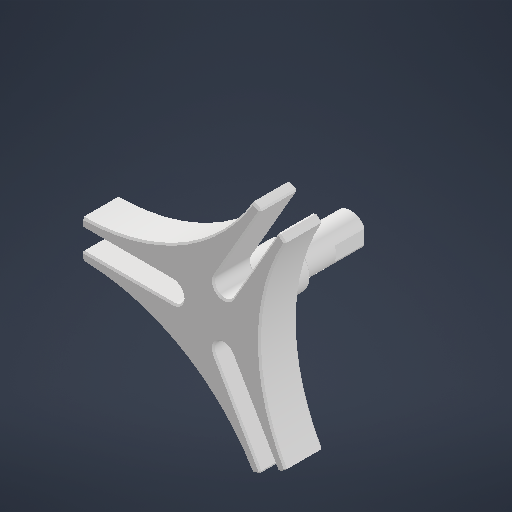
# Autodesk Inventor part: Geneva2_Output
Saved by Autodesk Inventor 2026.3 (Build 303398000, 398)
## iProperties
Created: 2026-05-01
Part Number: Geneva2_Output
Material: Generic
Document SubType Name: Modeling
Designer: frede
Density: 1 g/cm^3
Appearance: Default
Author: frede
Autodesk Inventor part; units mm, degrees
ref_plane "YZ Plane" through (0, 0, 0) normal (1, 0, 0) x (0, 1, 0)
ref_plane "XZ Plane" through (0, 0, 0) normal (0, 1, 0) x (-1, 0, 0)
ref_plane "XY Plane" through (0, 0, 0) normal (0, 0, 1) x (1, 0, 0)
sketch "Sketch2" plane through (0, 0, 0) normal (0, 0, 1) x (1, 0, 0)
  line L0 (0, 0) -> (10, 17.3205)
  line L1 (0, 0) -> (20, 0) construction
  line L2 (10, 17.3205) -> (40, 0)
  line L3 (0, 0) -> (40, 0)
  circle A0 centre (0, 0) radius 20
  circle A1 centre (40, 0) radius 34.641
  circle A2 centre (0, 0) radius 5.359
  arc A3 (1.2939, 5.441) -> (4.0651, 3.841) centre (2.6795, 4.641) ccw
  line L4 (8.4, 17.3205) -> (8.4, 0)
  arc A4 (8.4, 0) -> (12.518, -15.5981) centre (40, 0) ccw
  arc A5 (12.518, 15.5981) -> (8.4, 0) centre (40, 0) ccw
  arc A6 (12.518, -15.5981) -> (12.518, 15.5981) centre (40, 0) ccw
  line L5 (1.2939, 5.441) -> (8.6144, 18.1205)
  line L6 (11.3856, 16.5205) -> (4.0651, 3.841)
  arc A7 (11.3525, 16.4657) -> (8.5835, 18.0644) centre (10, 17.3205) ccw
  arc A8 (-19.7673, 3.0419) -> (-4.2, 7.2746) centre (-20, 34.641) ccw
  line L7 (-20, 1.6) -> (-5.359, 1.6)
  line L8 (-5.359, -1.6) -> (-20, -1.6)
  arc A9 (-5.359, -1.6) -> (-5.359, 1.6) centre (-5.359, 0) ccw
  arc A10 (-4.2, 7.2746) -> (7.2493, 18.6399) centre (-20, 34.641) ccw
  arc A11 (7.2493, -18.6399) -> (-4.2, -7.2746) centre (-20, -34.641) ccw
  line L9 (8.6144, -18.1205) -> (1.2939, -5.441)
  line L10 (4.0651, -3.841) -> (11.3856, -16.5205)
  arc A12 (4.0651, -3.841) -> (1.2939, -5.441) centre (2.6795, -4.641) ccw
  arc A13 (-4.2, -7.2746) -> (-19.7673, -3.0419) centre (-20, -34.641) ccw
  point P0 (0, 0)
  point P1 (8.5823, 18.065)
  point P2 (7.2493, 18.6399)
  point P3 (-19.7673, 3.0419)
  point P4 (-19.9359, 1.6)
  point P5 (-19.9359, -1.6)
  point P6 (-19.7673, -3.0419)
  point P7 (7.2493, -18.6399)
  point P8 (8.5823, -18.065)
  point P9 (11.3536, -16.465)
  point P10 (11.3536, 16.465)
  dimension "d2" = 20
  dimension "d3" = 60
  dimension "d4" = 3.2
  dimension "d5" = 360
  constraints: 27 point on circle, 22 end point, 12 centre point, 5 coincident, 5 tangent, 3 point on line, 2 perpendicular, 1 equal length, 1 horizontal, 49 other
  measures "d2" distance of L0.start L0.end
  measures "d3" angle of L1 L0
  measures "d4" diameter of A3
extrude "Extrusion1" add sketch "Sketch2" along normal blind 6 contours L3 A2 A12 A9 A3 L0 | L0 A3 A2 L3 | A1 L6 L4 L3 | A2 A3 L6 A1 | L3 A4 A0 L10 A1 | A1 L10 A12 A2 | A2 A9 L7 A0 A8 A10 L5 A3 | L4 L6 A0 A5 | A12 L9 A0 A11 A13 L8 A9 A2
sketch "Sketch3" plane through (0, 0, 0) normal (0, 0, -1) x (-1, 0, 0)
  circle A0 centre (0, 0) radius 3.5
  dimension "d9" = 7
  constraints: 1 centre point, 1 coincident
  measures "d9" diameter of A0
extrude "Extrusion2" add sketch "Sketch3" along normal blind 7.1
sketch "Sketch4" plane through (0, 0, -7.1) normal (0, 0, -1) x (-1, 0, 0)
  circle A0 centre (0, 0) radius 3.5 projected
  circle A1 centre (0, 0) radius 2.5
  dimension "d12" = 5
  constraints: 1 centre point, 1 coincident
  measures "d12" diameter of A1
extrude "Extrusion3" add sketch "Sketch4" along normal blind 10 contours A1
fillet "Fillet1" radius 0.4 2 edges at (2.5, 0, -7.1) (3.5, 0, 0)
sketch "Sketch5" plane through (0, 0, -17.1) normal (0, 0, -1) x (-1, 0, 0)
  circle A0 centre (0, 0) radius 2.5 projected
  line L0 (-2.25, -1.0897) -> (-2.25, 1.0897)
  dimension "d19" = 2.25
  constraints: 2 end point, 2 point on circle, 1 vertical
  measures "d19" distance from line of point (0, 0) L0
extrude "Extrusion4" cut sketch "Sketch5" against normal blind 5 contours L0 A0 picked at (-2.3122, 0.1863)
chamfer "Chamfer2" distance 0.25 angle 45 4 edges at (2.25, 0, -17.1) (-0.559, -2.4367, -17.1) (-0.559, 2.4367, -17.1) (3.5, 0, -7.1)
chamfer "Chamfer3" distance 0.25 angle 45 49 edges at (8.4, 0, 6) (11.9437, -16.0421, 6) (7.7094, -10.153, 6) (1.8795, -3.2554, 6) (4.9381, -11.753, 6) (7.921, -18.3646, 6) (-4.2, -7.2746, 6) (-12.6474, -1.6, 6) (-3.759, 0, 6) (-12.6474, 1.6, 6) (-4.2, 7.2746, 6) (1.8795, 3.2554, 6) (4.9381, 11.753, 6) (7.7094, 10.153, 6) (7.921, 18.3646, 6) (11.9437, 16.0421, 6) (-19.8647, -2.3225, 6) (-19.8647, 2.3225, 6) (7.7094, -10.153, 0) (3.3613, -3.1935, 0) (1.8795, -3.2554, 0) (1.0851, -4.5077, 0) (4.9381, -11.753, 0) (11.9437, -16.0421, 0) (8.4, 0, 0) (7.7094, 10.153, 0) (3.3613, 3.1935, 0) (1.8795, 3.2554, 0) (1.0851, 4.5077, 0) (4.9381, 11.753, 0) (11.9437, 16.0421, 0) (7.921, 18.3646, 0) (-4.2, 7.2746, 0) (-19.8647, 2.3225, 0) (-12.6474, 1.6, 0) (-4.4463, 1.3142, 0) (-3.7823, 0.2724, 0) (-3.7823, -0.2724, 0) (-4.4463, -1.3142, 0) (-12.6474, -1.6, 0) (-19.8647, -2.3225, 0) (-4.2, -7.2746, 0) (7.921, -18.3646, 0) (8.5823, -18.065, 3) (11.3536, -16.465, 3) (-19.9359, -1.6, 3) (-19.9359, 1.6, 3) (8.5823, 18.065, 3) (11.3536, 16.465, 3)
equation "\"d4\" = d6"
equation "\"d6\" = 3.2"
body "Solid1"
